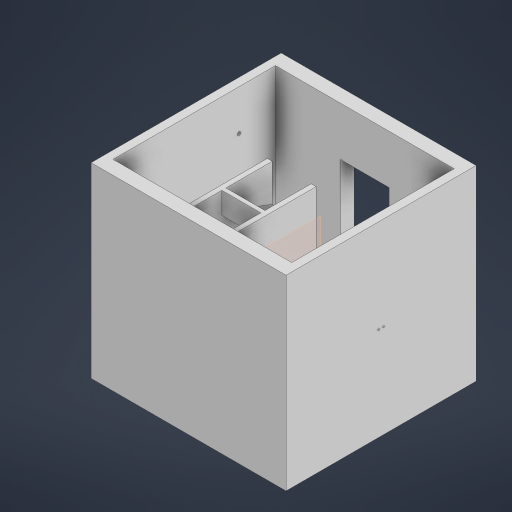
# Autodesk Inventor part: shooter-comp
Saved by Autodesk Inventor 2023 (Build 270158000, 158)
## iProperties
Created: 2022-05-15
Part Number: shooter-comp
Material: Generic
Document SubType Name: Modeling
Designer: jayso
Density: 1 g/cm^3
Appearance: Default
Author: jayso
Autodesk Inventor part; units mm, degrees
ref_plane "YZ Plane" through (0, 0, 0) normal (1, 0, 0) x (0, 1, 0)
ref_plane "XZ Plane" through (0, 0, 0) normal (0, 1, 0) x (-1, 0, 0)
ref_plane "XY Plane" through (0, 0, 0) normal (0, 0, 1) x (1, 0, 0)
sketch "Sketch2" plane through (0, 0, 0) normal (0, 1, 0) x (-1, 0, 0)
  line L0 (60, 58.5) -> (-60, 58.5)
  line L1 (-60, 58.5) -> (-60, -58.5)
  line L2 (-60, -58.5) -> (60, -58.5)
  line L3 (60, -58.5) -> (60, 58.5)
  point P0 (0, 0)
  dimension "d0" = 117
  dimension "d1" = 120
  dimension "d2" = 58.5
  dimension "d3" = 60
  constraints: 8 end point, 2 parallel, 1 horizontal, 1 perpendicular
  measures "d0" distance between parallel lines of L2 L0
  measures "d1" distance of L1.end L2.end
  measures "d2" vertical distance of point (0, 0) L2.end
  measures "d3" horizontal distance of point (0, 0) L0.start
extrude "Extrusion1" add sketch "Sketch2" along normal blind 115
sketch "Sketch3" plane through (-60, 0, -58.5) normal (-1, 0, 0) x (0, 0, 1)
  circle A0 centre (58.5, 57.5) radius 4
  line L0 (0, 115) -> (117, 115) projected
  line L1 (0, 0) -> (0, 115) projected
  point P0 (58.5, 0)
  point P1 (58.5, 115)
  dimension "d6" = 8
  dimension "d7" = 57.5
  dimension "d8" = 58.5
  constraints: 1 centre point, 1 midpoint
  measures "d6" diameter of A0
  measures "d7" distance of point (58.5, 115) A0.centre
  measures "d8" distance from line of L1 A0.centre
extrude "Extrusion2" add sketch "Sketch3" along normal blind 34
sketch "Sketch4" plane through (0, 115, 0) normal (0, 1, 0) x (1, 0, 0)
  line L0 (-55, 50) -> (55, 50)
  line L1 (55, 50) -> (55, -50)
  line L2 (55, -50) -> (-55, -50)
  line L3 (-55, -50) -> (-55, 50)
  line L4 (-60, 58.5) -> (-60, -58.5) projected
  line L5 (-60, -58.5) -> (60, -58.5) projected
  point P0 (0, 0)
  dimension "d11" = 110
  dimension "d12" = 5
  dimension "d13" = 100
  dimension "d14" = 8.5
  constraints: 8 end point, 2 parallel, 1 horizontal, 1 perpendicular
  measures "d11" distance of L0.start L0.end
  measures "d12" distance between parallel lines of L4 L3
  measures "d13" distance of L0.end L1.end
  measures "d14" distance from line of L5 L1.end
extrude "Extrusion3" cut sketch "Sketch4" against normal blind 110
sketch "Sketch12" plane through (60, 0, 58.5) normal (1, 0, 0) x (0, 0, -1)
  circle A0 centre (58.5, 57.5) radius 4 projected
  circle A1 centre (57, 57.5) radius 0.5
  circle A2 centre (60, 57.5) radius 0.5
  point P0 (58.5, 0)
  point P1 (54.5, 57.5)
  point P2 (62.5, 57.5)
  point P3 (57.5, 57.5)
  point P4 (59.5, 57.5)
  dimension "d34" = 1
  dimension "d35" = 1
  dimension "d36" = 2
  dimension "d38" = 2.5
  dimension "d39" = 2.5
  constraints: 2 horizontal alignment, 2 point on circle, 4 other
  measures "d36" distance of point (59.5, 57.5) point (57.5, 57.5)
  measures "d38" distance of A0.start point (57, 57.5)
  measures "d39" distance of A0.end point (60, 57.5)
extrude "Extrusion6" cut sketch "Sketch12" against normal blind 5 contours A1 | A2
sketch "Sketch13" plane through (55, 115, 50) normal (0, 0, -1) x (-1, 0, 0)
  line L0 (40, -28) -> (70, -28)
  line L1 (70, -28) -> (70, -110)
  line L2 (70, -110) -> (40, -110)
  line L3 (40, -110) -> (40, -28)
  line L4 (0, 0) -> (110, 0) projected
  line L5 (0, -110) -> (110, -110) projected
  point P0 (55, -115)
  point P1 (55, 0)
  point P2 (70, -69)
  point P3 (40, -69)
  point P4 (55, -110)
  dimension "d44" = 28
  dimension "d45" = 40
  dimension "d46" = 40
  dimension "d47" = 0
  constraints: 8 end point, 4 midpoint, 2 parallel, 1 horizontal, 1 perpendicular
  measures "d44" distance from line of point (55, 0) L0
  measures "d45" horizontal distance of L4.end point (70, -69)
  measures "d46" horizontal distance of L4.start point (40, -69)
  measures "d47" distance from line of point (55, -110) L2
sketch "Sketch14" plane through (-55, 115, -50) normal (0, 0, 1) x (1, 0, 0)
  line L0 (0, -110) -> (110, -110) projected
  line L1 (40, -110) -> (70, -110)
  line L2 (70, -110) -> (70, -80)
  line L3 (70, -80) -> (40, -80)
  line L4 (40, -80) -> (40, -110)
  line L5 (0, 0) -> (0, -110) projected
  line L6 (110, 0) -> (110, -110) projected
  point P0 (55, -115)
  point P1 (40, -95)
  point P2 (70, -95)
  dimension "d48" = 40
  dimension "d49" = 40
  dimension "d50" = 30
  constraints: 8 end point, 2 midpoint, 2 parallel, 1 horizontal, 1 perpendicular, 1 point on line
  measures "d48" distance from line of L5 point (40, -95)
  measures "d49" distance from line of L6 point (70, -95)
  measures "d50" distance of L1.end L2.end
loft "Loft1" add profiles "Sketch13", "Sketch14"
sketch "Sketch18" plane through (-15, 5, 50) normal (-1, 0, 0) x (0, 0, 1)
  line L0 (-100, 0) -> (-100, 30) projected
  line L1 (-100, 0) -> (-55, 0)
  line L2 (0, 0) -> (-100, 0) projected
  line L3 (-55, 0) -> (-55, 53.4)
  line L4 (0, 82) -> (-100, 30) projected
  line L5 (-55, 53.4) -> (-105.2382, 30.2966)
  point P0 (-50, -5)
  dimension "d57" = 45
  constraints: 6 end point, 2 point on line, 1 perpendicular
  measures "d57" distance of L0.start L1.end
extrude "Extrusion7" cut sketch "Sketch18" against normal blind 30
ref_plane "Work Plane2" through (15, 5, 50) normal (1, 0, 0) x (0, 0, -1)
sketch "Sketch28" plane through (15, 5, 50) normal (1, 0, 0) x (0, 0, -1)
  line L0 (55, 0) -> (55, 53.4) projected
  line L1 (55, 53.4) -> (55, 118.4)
  line L2 (55, 53.4) -> (55, 0) projected
  line L3 (55, 118.4) -> (0, 118.4)
  line L4 (0, 82) -> (55, 53.4) projected
  line L5 (0, 118.4) -> (0, 82)
  line L6 (0, 82) -> (55, 53.4)
  point P0 (50, -5)
  dimension "d75" = 65
  constraints: 8 end point, 2 perpendicular, 1 collinear
  measures "d75" distance of L0.end L1.end
extrude "Extrusion8" add sketch "Sketch28" against normal blind 3
ref_plane "Work Plane3" through (-15, 5, 50) normal (-1, 0, 0) x (0, 0, 1)
sketch "Sketch31" plane through (-15, 5, 50) normal (-1, 0, 0) x (0, 0, 1)
  line L0 (0, 82) -> (-55, 53.4) projected
  line L1 (-55, 53.4) -> (-55, 117.6573)
  line L2 (-55, 0) -> (-55, 118.4) projected
  line L3 (-55, 118.4) -> (0, 118.4)
  line L4 (0, 118.4) -> (0, 82)
  point P0 (-50, -5)
  constraints: 6 end point, 1 horizontal, 1 perpendicular, 1 vertical
extrude "Extrusion9" add sketch "Sketch31" against normal blind 3
sketch "Sketch32" plane through (-15, 5, -5) normal (-1, 0, 0) x (0, 0, 1)
  line L0 (0, 0) -> (0, 118.4) projected
  line L1 (0, 118.4) -> (55, 118.4)
  line L2 (55, 118.4) -> (55, 103)
  line L3 (55, 103) -> (0, 103)
  line L4 (0, 103) -> (0, 118.4)
  point P0 (5, -5)
  point P1 (0, 103)
  dimension "d81" = 15.4
  constraints: 8 end point, 2 parallel, 1 horizontal, 1 perpendicular
  measures "d81" distance of L1.end L2.end
extrude "Extrusion10" cut sketch "Sketch32" against normal blind 30
sketch "Sketch33" plane through (-55, 115, 50) normal (1, 0, 0) x (0, 0, -1)
  circle A0 centre (77.5, -73) radius 14
  circle A1 centre (77.5, -25) radius 14
  line L0 (0, 0) -> (100, 0) projected
  line L1 (77.5, -39) -> (77.5, -59)
  line L2 (100, 0) -> (100, -110) projected
  circle A2 centre (77.5, -73) radius 1
  circle A3 centre (77.5, -25) radius 1
  point P0 (50, -115)
  dimension "d84" = 28
  dimension "d85" = 28
  dimension "d86" = 48
  dimension "d101" = 25
  dimension "d102" = 22.5
  dimension "d130" = 2
  dimension "d131" = 2
  constraints: 2 centre point, 2 coincident, 2 end point, 2 vertical alignment, 1 vertical, 4 other
  measures "d86" distance of point (77.5, -73) point (77.5, -25)
  measures "d101" distance from line of L0 point (77.5, -25)
  measures "d102" distance from line of L2 point (77.5, -25)
  measures "d130" diameter of A2
  measures "d131" diameter of A3
sketch "Sketch43" plane through (60, 0, -58.5) normal (0, 0, -1) x (-1, 0, 0)
  line L0 (45, 5) -> (45, 108) projected
  line L1 (75, 108) -> (75, 5) projected
  line L2 (45, 85) -> (75, 85)
  line L3 (75, 85) -> (75, 30)
  line L4 (75, 30) -> (45, 30)
  line L5 (45, 30) -> (45, 85)
  line L6 (0, 115) -> (120, 115) projected
  line L7 (0, 0) -> (120, 0) projected
  point P0 (60, 0)
  point P1 (45, 30)
  point P2 (75, 85)
  point P3 (60, 115)
  point P4 (60, 85)
  point P5 (60, 0)
  dimension "d119" = 30
  dimension "d120" = 30
  constraints: 8 end point, 3 midpoint, 2 parallel, 2 point on line, 1 horizontal, 1 perpendicular
  measures "d119" distance of point (60, 115) point (60, 85)
  measures "d120" distance from line of point (60, 0) L4
extrude "Extrusion17" cut sketch "Sketch43" against normal blind 8.5
sketch "Sketch44" plane through (-15, 5, -5) normal (-1, 0, 0) x (0, 0, 1)
  line L0 (0, 103) -> (55, 103) projected
  line L1 (31, 91.6613) -> (0, 80)
  line L2 (0, 103) -> (0, 53.4) projected
  line L3 (55, 103) -> (55, 101)
  line L4 (31, 89.6613) -> (0, 78)
  line L5 (0, 78) -> (0, 80)
  line L6 (31, 91.6613) -> (31, 89.6613)
  point P0 (5, -5)
  dimension "d121" = 2
  dimension "d125" = 23
  dimension "d126" = 2
  constraints: 10 end point, 2 point on line, 2 vertical, 1 parallel
  measures "d121" distance of L0.end L3.end
  measures "d125" distance of L0.start L1.end
  measures "d126" distance of L1.end L4.end
extrude "Extrusion18" add sketch "Sketch44" against normal blind 30
sketch "Sketch46" plane through (12, 5, 50) normal (-1, 0, 0) x (0, 0, 1)
  line L0 (-55, 80) -> (-24, 91.6613) projected
  line L1 (-26.5, 90.7209) -> (-24, 91.6613)
  line L2 (-24, 91.6613) -> (-24, 103)
  line L3 (0, 103) -> (-55, 103) projected
  line L4 (-26.5, 103) -> (-26.5, 90.7209)
  point P0 (-50, -5)
  dimension "d127" = 2.5
  constraints: 6 end point, 3 point on line, 1 collinear, 1 parallel, 1 vertical
  measures "d127" distance between parallel lines of L2 L4
extrude "Extrusion19" add sketch "Sketch46" along normal blind 27
extrude "Extrusion20" cut sketch "Sketch33" against normal blind 5 contours A2 | A3
body "Solid1"
